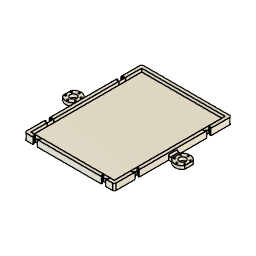
ElevatorAssembly (Autodesk Fusion 360 archive; units mm, degrees)
design "lift_platform"
part number: 2025-09-29-11-11-04-604
Autodesk Fusion 360 part; units mm, degrees
(part 1 of 2)
sketch "Sketch8" plane through (0, 0, 0) normal (0, 0, 1) x (1, 0, 0)
  line L0 (0, 0) -> (256, 0)
  line L1 (256, 0) -> (256, 340)
  line L2 (256, 340) -> (0, 340)
  line L3 (0, 340) -> (0, 0)
  line L4 (0, 340) -> (256, 340)
  line L5 (256, 340) -> (256, 350)
  line L6 (256, 350) -> (0, 350)
  line L7 (0, 350) -> (0, 340)
  line L8 (0, 350) -> (-10, 350)
  line L9 (-10, 350) -> (-10, 0)
  line L10 (-10, 0) -> (0, 0)
  line L11 (0, 0) -> (0, 350)
  line L12 (-10, 0) -> (256, 0)
  line L13 (256, 0) -> (256, -10)
  line L14 (256, -10) -> (-10, -10)
  line L15 (-10, -10) -> (-10, 0)
  line L16 (256, 350) -> (266, 350)
  line L17 (266, 350) -> (266, -10)
  line L18 (266, -10) -> (256, -10)
  line L19 (256, -10) -> (256, 350)
  line L20 (0, 170) -> (256, 170)
  line L21 (256, 170) -> (276, 170)
  line L22 (276, 170) -> (276, 156.885)
  line L23 (276, 156.885) -> (256, 156.885)
  line L24 (256, 156.885) -> (256, 170)
  line L25 (256, 170) -> (276, 170)
  line L26 (276, 170) -> (276, 183.115)
  line L27 (276, 183.115) -> (256, 183.115)
  line L28 (256, 183.115) -> (256, 170)
  line L29 (128, 340) -> (128, 0)
  line L30 (-20, 170) -> (-20, 156.885)
  line L31 (0, 170) -> (-20, 170)
  line L32 (-20, 156.885) -> (0, 156.885)
  line L33 (0, 183.115) -> (0, 170)
  line L34 (-20, 170) -> (-20, 183.115)
  line L35 (0, 170) -> (-20, 170)
  line L36 (0, 156.885) -> (0, 170)
  line L37 (-20, 183.115) -> (0, 183.115)
  dimension "d58" = 340
  dimension "d59" = 256
  dimension "d60" = 10
  dimension "d61" = 10
  dimension "d62" = 10
  dimension "d63" = 10
  dimension "d64" = 20
  dimension "d65" = 13.115
  dimension "d66" = 13.115
  constraint horizontal L0
  constraint vertical L1
  constraint horizontal L2
  constraint vertical L3
  constraint coincident L0.start L3.end
  constraint horizontal L4
  constraint vertical L5
  constraint horizontal L6
  constraint vertical L7
  constraint horizontal L8
  constraint vertical L9
  constraint horizontal L10
  constraint vertical L11
  constraint horizontal L12
  constraint vertical L13
  constraint horizontal L14
  constraint vertical L15
  constraint horizontal L16
  constraint vertical L17
  constraint horizontal L18
  constraint vertical L19
  constraint midpoint L3 L20.start
  constraint midpoint L19 L20.end
  constraint perpendicular L19 L20
  constraint horizontal L21
  constraint vertical L22
  constraint horizontal L23
  constraint vertical L24
  constraint horizontal L25
  constraint vertical L26
  constraint horizontal L27
  constraint vertical L28
  constraint midpoint L2 L29.start
  constraint midpoint L0 L29.end
  constraint symmetric L20.end L29 L20.start
  constraint symmetric L21.end L29 L30.start
  constraint symmetric L22.end L29 L30.end
  constraint symmetric L23.end L29 L32.end
  constraint symmetric L26.end L29 L34.end
  constraint symmetric L27.end L29 L33.start
  measures "d58" distance of L0.start L2.end
  measures "d59" distance of L0.start L0.end
  measures "d60" distance of L2.end L6.end
  measures "d61" distance of L6.end L8.end
  measures "d62" distance of L9.end L14.end
  measures "d63" distance of L5.end L16.end
  measures "d64" distance of L20.end L21.end
  measures "d65" distance of L20.end L23.end
  measures "d66" distance of L20.end L27.end
extrude "Extrude10" add sketch "Sketch8" along normal blind 15 makes body 1
sketch "Sketch9" plane through (0, 0, 15) normal (0, 0, 1) x (-1, 0, 0)
  line L0 (20, -183.115) -> (20, -156.885)
  line L1 (20, -156.885) -> (10, -156.885)
  line L2 (10, -156.885) -> (10, 10)
  line L3 (10, 10) -> (-266, 10)
  line L4 (-266, 10) -> (-266, -156.885)
  line L5 (-266, -156.885) -> (-276, -156.885)
  line L6 (-276, -156.885) -> (-276, -183.115)
  line L7 (-276, -183.115) -> (-266, -183.115)
  line L8 (-266, -183.115) -> (-266, -350)
  line L9 (-266, -350) -> (10, -350)
  line L10 (10, -350) -> (10, -183.115)
  line L11 (10, -183.115) -> (20, -183.115)
  line L12 (-256, -156.885) -> (-256, -170)
  line L13 (-128, 0) -> (-128, -340)
  line L14 (-256, 10) -> (-256, 0)
  line L15 (-266, -340) -> (-256, -340)
  line L16 (0, -340) -> (0, 0)
  line L17 (-256, -340) -> (0, -340)
  line L18 (0, 0) -> (-256, 0)
  line L19 (-266, -340) -> (0, -340)
  line L20 (0, -350) -> (-266, -350)
  line L21 (-256, 0) -> (-256, -340)
  line L22 (-266, -350) -> (-266, -340)
  line L23 (0, -350) -> (0, 10)
  line L24 (-256, -170) -> (-276, -170)
  line L25 (-256, -183.115) -> (-256, -170)
  line L26 (10, 10) -> (10, -350)
  line L27 (-276, -170) -> (-276, -183.115)
  line L28 (-276, -183.115) -> (-256, -183.115)
  line L29 (0, -156.885) -> (0, -170)
  line L30 (10, -350) -> (0, -350)
  line L31 (0, 10) -> (10, 10)
  line L32 (20, -183.115) -> (0, -183.115)
  line L33 (-256, -340) -> (-256, 10)
  line L34 (-276, -156.885) -> (-256, -156.885)
  line L35 (-276, -170) -> (-276, -156.885)
  line L36 (0, 0) -> (0, 10)
  line L37 (0, -183.115) -> (0, -170)
  line L38 (20, -170) -> (20, -156.885)
  line L39 (-266, 10) -> (-266, -340)
  line L40 (-256, 10) -> (-266, 10)
  line L41 (0, -340) -> (0, -350)
  line L42 (0, -170) -> (20, -170)
  line L43 (20, -156.885) -> (0, -156.885)
  line L44 (20, -170) -> (20, -183.115)
  line L45 (-256, -170) -> (-276, -170)
  line L46 (0, -170) -> (20, -170)
  line L47 (-256, -170) -> (0, -170)
  line L48 (-256, 0) -> (0, 0)
  line L49 (0, 10) -> (-256, 10)
  point P0 (-256, -340)
  dimension "d69" = 340
  dimension "d70" = 256
  dimension "d71" = 10
  dimension "d72" = 10
  dimension "d73" = 10
  dimension "d74" = 10
  dimension "d75" = 20
  dimension "d76" = 13.115
  dimension "d77" = 13.115
  constraint horizontal L17
  constraint vertical L16
  constraint horizontal L18
  constraint vertical L21
  constraint coincident P0 L15.end
  constraint horizontal L48
  constraint vertical L36
  constraint horizontal L49
  constraint vertical L14
  constraint horizontal L40
  constraint vertical L39
  constraint horizontal L15
  constraint vertical L33
  constraint horizontal L19
  constraint vertical L41
  constraint horizontal L20
  constraint vertical L22
  constraint horizontal L31
  constraint vertical L26
  constraint horizontal L30
  constraint vertical L23
  constraint midpoint L12.end L21
  constraint midpoint L29.end L23
  constraint perpendicular L23 L47
  constraint horizontal L46
  constraint vertical L44
  constraint horizontal L32
  constraint vertical L37
  constraint horizontal L42
  constraint vertical L38
  constraint horizontal L43
  constraint vertical L29
  constraint midpoint L13.start L18
  constraint midpoint L13.end L17
  constraint symmetric L12.end L29.end L13
  constraint symmetric L24.end L38.start L13
  constraint symmetric L0.start L6.end L13
  constraint symmetric L32.end L25.start L13
  constraint symmetric L38.start L24.end L13
  constraint symmetric L5.end L0.end L13
  constraint symmetric L12.start L29.start L13
  measures "d69" distance of P0 L14.end
  measures "d70" distance of L16.start P0
  measures "d71" distance of L14.end L14.start
  measures "d72" distance of L3.end L14.start
  measures "d73" distance of L15.start L8.end
  measures "d74" distance of L2.end L23.end
  measures "d75" distance of L38.start L29.end
  measures "d76" distance of L32.end L29.end
  measures "d77" distance of L29.start L29.end
extrude "Extrude11" add sketch "Sketch9" along normal blind 10 contours L16 L23 L26 L32 L37 L42 L46 | L9 L10 L16 L23 L26 L30 L32 L41 | L16 L23 L26 L29 L42 L43 L46 | L2 L3 L16 L23 L26 L31 L36 L43 | L8 L9 L15 L17 L19 L20 L22 L23 L41 | L3 L14 L18 L23 L33 L36 L48 L49 | L12 L21 L24 L33 L34 L39 L45 | L21 L24 L25 L28 L33 L39 L45 | L8 L15 L19 L21 L28 L33 L39 | L3 L4 L14 L21 L33 L34 L39 L40 bodies 1
sketch "Sketch10" plane through (0, 0, 15) normal (0, 0, 1) x (-1, 0, 0)
  line L0 (0, -340) -> (0, 0)
  line L1 (0, 0) -> (-256, 0)
  line L2 (-256, 0) -> (-256, -340)
  line L3 (-256, -340) -> (0, -340)
  arc A0 (109.5, -146.8851) -> (70.5, -146.8851) centre (90, -160) ccw
  circle A1 centre (105.1554, -168.75) radius 2.5
  line L4 (109.5, -173.1149) -> (109.5, -146.8851)
  circle A2 centre (90, -160) radius 10
  line L5 (90, -136.5) -> (90, -183.5)
  line L6 (70.5, -146.8851) -> (70.5, -173.1149)
  line L7 (109.5, -173.1149) -> (109.5, -146.8851)
  line L8 (70.5, -146.8851) -> (70.5, -172.6262)
  circle A3 centre (90, -142.5) radius 2.5
  circle A4 centre (74.8446, -151.25) radius 2.5
  circle A5 centre (74.8446, -168.75) radius 2.5
  arc A6 (70.5, -173.1149) -> (109.5, -173.1149) centre (90, -160) ccw
  circle A7 centre (90, -160) radius 11
  circle A8 centre (105.1554, -151.25) radius 2.5
  circle A9 centre (90, -177.5) radius 2.5
  point P0 (90, -160)
  constraint coincident L4.start L7.start
  constraint coincident A0.start L4.end
  constraint coincident A0.end L6.start
  constraint coincident L8.end L6
  constraint midpoint L5.start A0
  constraint midpoint L5.end A6
  constraint concentric A2 A6
extrude "Extrude12" add sketch "Sketch10" along normal blind 15 separate body contours A0 L4 L5 L7 A3 A6 A7 A9 | A0 L5 L6 L8 A3 A6 A7 A9 | A2 L5 A7 | A2 L5 A7 makes body 2
extrude "Extrude13" cut 3 faces at (85.3333, 226.6667, 15) (-13.3333, 165.6283, 15) (269.3333, 174.3717, 15) along direction (0, 0, -1) blind 5 on bodies 1 bodies 1
extrude "Extrude14" cut 1 faces at (262.6667, 226.6667, 25) along direction (0, 0, -1) blind 5 on bodies 1 bodies 1
extrude "Extrude15" cut 1 faces at (-80.6272, 175.6522, 30) along direction (0, 0, -1) blind 5 on bodies 2 bodies 2
copy_body "CopyPasteBodies2" bodies 2 makes body 3
move_body "Move2" bodies 3 to x (1, 0, 0) y (0, 1, 0) z (0, 0, 1) at (440, 0, 0)
move_body "Align1" bodies 2 to x (1, 0, 0) y (0, 1, 0) z (0, 0, 1) at (50.5, 10, -15)
move_body "Align2" bodies 3 to x (1, 0, 0) y (0, 1, 0) z (0, 0, 1) at (-54.5, 10, -15)
fillet "Fillet4" radius 5 4 edges at (-10, -10, 10) (266, -10, 10) (266, 350, 10) (-10, 350, 10) on bodies 1
fillet "Fillet5" radius 5 2 edges at (266, 170, 10) (-10, 170, 10) on bodies 1
sketch "Sketch11" plane through (0, 0, 20) normal (0, 0, 1) x (-1, 0, 0)
  line L0 (0, -340) -> (-256, -340)
  line L1 (-256, -340) -> (-256, 0)
  line L2 (-256, 0) -> (0, 0)
  line L3 (0, 0) -> (0, -340)
  arc A0 (5, -350) -> (10, -345) centre (5, -345) ccw
  line L4 (10, -345) -> (10, 5)
  arc A1 (10, 5) -> (5, 10) centre (5, 5) ccw
  line L5 (5, 10) -> (-261, 10)
  arc A2 (-261, 10) -> (-266, 5) centre (-261, 5) ccw
  line L6 (-266, 5) -> (-266, -345)
  arc A3 (-266, -345) -> (-261, -350) centre (-261, -345) ccw
  line L7 (-261, -350) -> (5, -350)
  line L8 (-128, 10) -> (-128, -350)
  line L9 (-324.6319, -170) -> (70, -170)
  line L10 (-13, 0.0014) -> (-33, 0.0014)
  line L11 (-33, 0.0014) -> (-33, 7)
  line L12 (-33, 0.0014) -> (-33, 7)
  line L13 (-13, 7) -> (-13, 0.0014)
  line L14 (-13, 0.0014) -> (-33, 0.0014)
  line L15 (-13, 7) -> (-13, 0.0014)
  line L16 (-33, 7) -> (-13, 7)
  line L17 (-33, 7) -> (-13, 7)
  line L18 (7, -49.9986) -> (7, -69.9986)
  line L19 (7, -69.9986) -> (0.0014, -69.9986)
  line L20 (7, -69.9986) -> (0.0014, -69.9986)
  line L21 (0.0014, -49.9986) -> (7, -49.9986)
  line L22 (7, -49.9986) -> (7, -69.9986)
  line L23 (0.0014, -49.9986) -> (7, -49.9986)
  line L24 (0.0014, -69.9986) -> (0.0014, -49.9986)
  line L25 (0.0014, -69.9986) -> (0.0014, -49.9986)
  line L26 (-33, 7) -> (-13, 7)
  line L27 (-13, 7) -> (-13, 10)
  line L28 (-13, 10) -> (-33, 10)
  line L29 (-33, 10) -> (-33, 7)
  line L30 (7, -49.9986) -> (10, -49.9986)
  line L31 (10, -49.9986) -> (10, -69.9986)
  line L32 (10, -69.9986) -> (7, -69.9986)
  line L33 (7, -69.9986) -> (7, -49.9986)
  line L34 (-33, 10) -> (-29, 10)
  line L35 (-29, 10) -> (-29, 7)
  line L36 (-29, 7) -> (-33, 7)
  line L37 (-33, 7) -> (-33, 10)
  line L38 (-13, 10) -> (-17, 10)
  line L39 (-17, 10) -> (-17, 7)
  line L40 (-17, 7) -> (-13, 7)
  line L41 (-13, 7) -> (-13, 10)
  line L42 (10, -49.9986) -> (7, -49.9986)
  line L43 (7, -49.9986) -> (7, -53.9986)
  line L44 (7, -53.9986) -> (10, -53.9986)
  line L45 (10, -53.9986) -> (10, -49.9986)
  line L46 (7, -69.9986) -> (10, -69.9986)
  line L47 (10, -69.9986) -> (10, -65.9986)
  line L48 (10, -65.9986) -> (7, -65.9986)
  line L49 (7, -65.9986) -> (7, -69.9986)
  line L50 (-263, -69.9986) -> (-256.0014, -69.9986)
  line L51 (-263, -69.9986) -> (-256.0014, -69.9986)
  line L52 (-256.0014, -49.9986) -> (-263, -49.9986)
  line L53 (-263, -49.9986) -> (-263, -69.9986)
  line L54 (-256.0014, -49.9986) -> (-263, -49.9986)
  line L55 (-256.0014, -69.9986) -> (-256.0014, -49.9986)
  line L56 (-256.0014, -69.9986) -> (-256.0014, -49.9986)
  line L57 (-263, -65.9986) -> (-263, -69.9986)
  line L58 (-263, -49.9986) -> (-263, -69.9986)
  line L59 (-266, -69.9986) -> (-266, -65.9986)
  line L60 (-263, -49.9986) -> (-263, -53.9986)
  line L61 (-266, -69.9986) -> (-263, -69.9986)
  line L62 (-263, -53.9986) -> (-266, -53.9986)
  line L63 (-266, -53.9986) -> (-266, -49.9986)
  line L64 (-266, -65.9986) -> (-263, -65.9986)
  line L65 (-263, -69.9986) -> (-266, -69.9986)
  line L66 (-266, -49.9986) -> (-266, -69.9986)
  line L67 (-266, -49.9986) -> (-263, -49.9986)
  line L68 (-263, -69.9986) -> (-263, -49.9986)
  line L69 (-263, -49.9986) -> (-266, -49.9986)
  line L70 (-223, 10) -> (-227, 10)
  line L71 (-227, 10) -> (-227, 7)
  line L72 (-239, 10) -> (-239, 7)
  line L73 (-239, 7) -> (-243, 7)
  line L74 (-243, 10) -> (-223, 10)
  line L75 (-223, 7) -> (-243, 7)
  line L76 (-243, 10) -> (-239, 10)
  line L77 (-227, 7) -> (-223, 7)
  line L78 (-243, 7) -> (-243, 0.0014)
  line L79 (-243, 7) -> (-243, 0.0014)
  line L80 (-223, 7) -> (-243, 7)
  line L81 (-243, 7) -> (-243, 10)
  line L82 (-223, 10) -> (-223, 7)
  line L83 (-243, 0.0014) -> (-223, 0.0014)
  line L84 (-223, 0.0014) -> (-223, 7)
  line L85 (-243, 7) -> (-243, 10)
  line L86 (-223, 7) -> (-223, 10)
  line L87 (-243, 0.0014) -> (-223, 0.0014)
  line L88 (-223, 0.0014) -> (-223, 7)
  line L89 (-223, 7) -> (-243, 7)
  line L90 (-243, -347) -> (-243, -340.0014)
  line L91 (-263, -270.0014) -> (-266, -270.0014)
  line L92 (-263, -290.0014) -> (-266, -290.0014)
  line L93 (-17, -347) -> (-13, -347)
  line L94 (-256.0014, -270.0014) -> (-256.0014, -290.0014)
  line L95 (-263, -290.0014) -> (-263, -286.0014)
  line L96 (-266, -286.0014) -> (-266, -290.0014)
  line L97 (-227, -347) -> (-223, -347)
  line L98 (-243, -347) -> (-243, -340.0014)
  line L99 (-223, -347) -> (-243, -347)
  line L100 (10, -290.0014) -> (7, -290.0014)
  line L101 (-13, -350) -> (-17, -350)
  line L102 (-243, -350) -> (-239, -350)
  line L103 (-263, -290.0014) -> (-263, -270.0014)
  line L104 (-263, -286.0014) -> (-266, -286.0014)
  line L105 (-243, -347) -> (-243, -350)
  line L106 (-33, -347) -> (-13, -347)
  line L107 (-239, -350) -> (-239, -347)
  line L108 (-239, -347) -> (-243, -347)
  line L109 (-13, -340.0014) -> (-33, -340.0014)
  line L110 (-13, -347) -> (-13, -340.0014)
  line L111 (7, -290.0014) -> (7, -270.0014)
  arc A4 (5, -350) -> (10, -345) centre (5, -345) ccw
  line L112 (7, -290.0014) -> (10, -290.0014)
  line L113 (-223, -340.0014) -> (-223, -347)
  line L114 (-223, -350) -> (-227, -350)
  line L115 (10, -270.0014) -> (10, -274.0014)
  line L116 (-13, -347) -> (-13, -350)
  line L117 (-33, -340.0014) -> (-33, -347)
  line L118 (7, -270.0014) -> (10, -270.0014)
  line L119 (-13, -347) -> (-13, -350)
  line L120 (7, -286.0014) -> (10, -286.0014)
  line L121 (-29, -350) -> (-29, -347)
  line L122 (-266, -270.0014) -> (-266, -274.0014)
  arc A5 (-266, -345) -> (-261, -350) centre (-261, -345) ccw
  line L123 (10, -290.0014) -> (10, -270.0014)
  line L124 (7, -270.0014) -> (7, -290.0014)
  line L125 (-13, -350) -> (-33, -350)
  line L126 (-243, -350) -> (-223, -350)
  line L127 (-256.0014, -270.0014) -> (-256.0014, -290.0014)
  line L128 (-266, -290.0014) -> (-263, -290.0014)
  line L129 (-33, -350) -> (-29, -350)
  line L130 (-13, -347) -> (-13, -340.0014)
  line L131 (7, -290.0014) -> (7, -286.0014)
  line L132 (-223, -347) -> (-243, -347)
  line L133 (-263, -274.0014) -> (-263, -270.0014)
  line L134 (-263, -290.0014) -> (-263, -270.0014)
  line L135 (-223, -347) -> (-243, -347)
  line L136 (-227, -350) -> (-227, -347)
  line L137 (-243, -340.0014) -> (-223, -340.0014)
  line L138 (-33, -347) -> (-13, -347)
  line L139 (10, -270.0014) -> (7, -270.0014)
  line L140 (-33, -340.0014) -> (-33, -347)
  line L141 (-29, -347) -> (-33, -347)
  line L142 (-33, -350) -> (-33, -347)
  line L143 (-263, -270.0014) -> (-263, -290.0014)
  line L144 (-243, -340.0014) -> (-223, -340.0014)
  line L145 (-266, -290.0014) -> (-266, -270.0014)
  line L146 (10, -274.0014) -> (7, -274.0014)
  line L147 (10, -286.0014) -> (10, -290.0014)
  line L148 (-33, -347) -> (-33, -350)
  line L149 (-243, -347) -> (-243, -350)
  line L150 (-266, -274.0014) -> (-263, -274.0014)
  line L151 (-266, -270.0014) -> (-263, -270.0014)
  line L152 (0.0014, -270.0014) -> (0.0014, -290.0014)
  line L153 (-223, -340.0014) -> (-223, -347)
  line L154 (-33, -347) -> (-13, -347)
  line L155 (-223, -347) -> (-223, -350)
  line L156 (0.0014, -270.0014) -> (0.0014, -290.0014)
  line L157 (-256.0014, -290.0014) -> (-263, -290.0014)
  line L158 (-223, -350) -> (-223, -347)
  line L159 (7, -274.0014) -> (7, -270.0014)
  line L160 (-13, -340.0014) -> (-33, -340.0014)
  line L161 (7, -290.0014) -> (7, -270.0014)
  line L162 (-17, -350) -> (-17, -347)
  line L163 (-263, -270.0014) -> (-256.0014, -270.0014)
  line L164 (-256, -340) -> (0, -340)
  line L165 (0.0014, -290.0014) -> (7, -290.0014)
  line L166 (0.0014, -290.0014) -> (7, -290.0014)
  line L167 (5, -350) -> (-261, -350)
  line L168 (7, -270.0014) -> (0.0014, -270.0014)
  line L169 (-263, -270.0014) -> (-256.0014, -270.0014)
  line L170 (7, -270.0014) -> (0.0014, -270.0014)
  line L171 (-256.0014, -290.0014) -> (-263, -290.0014)
  point P0 (-128, -350)
  point P1 (0, -340)
  dimension "d92" = 4
  dimension "d93" = 4
  constraint midpoint L5 L8.start
  constraint midpoint L7 P0
  constraint perpendicular L4 L9
  constraint horizontal L10
  constraint vertical L12
  constraint horizontal L16
  constraint vertical L13
  constraint horizontal L14
  constraint vertical L11
  constraint horizontal L17
  constraint vertical L15
  constraint horizontal L26
  constraint vertical L27
  constraint horizontal L28
  constraint vertical L29
  constraint coincident L5 L27.end
  constraint horizontal L30
  constraint vertical L31
  constraint horizontal L32
  constraint vertical L33
  constraint coincident L4 L31.end
  constraint horizontal L34
  constraint vertical L35
  constraint horizontal L36
  constraint vertical L37
  constraint coincident L16 L35.end
  constraint horizontal L38
  constraint vertical L39
  constraint horizontal L40
  constraint vertical L41
  constraint coincident L26 L39.end
  constraint horizontal L42
  constraint vertical L43
  constraint horizontal L44
  constraint vertical L45
  constraint horizontal L46
  constraint vertical L47
  constraint horizontal L48
  constraint vertical L49
  constraint symmetric L8 L10.start L78.end
  constraint symmetric L8 L13.start L73.end
  constraint symmetric L8 L11.end L75.start
  constraint symmetric L8 L10.end L83.end
  constraint symmetric L8 L18.start L52.end
  constraint symmetric L8 L21.start L52.start
  constraint symmetric L8 L19.end L50.end
  constraint symmetric L8 L18.end L50.start
  constraint symmetric L8 L27.end L74.start
  constraint symmetric L8 L28.end L70.start
  constraint symmetric L8 L30.end L63.end
  constraint symmetric L8 L31.end L59.start
  constraint symmetric L8 L34.end L70.end
  constraint symmetric L8 L35.end L71.end
  constraint symmetric L8 L38.end L72.start
  constraint symmetric L8 L39.end L72.end
  constraint symmetric L8 L43.end L60.end
  constraint symmetric L8 L44.end L62.end
  constraint symmetric L8 L47.end L59.end
  constraint symmetric L8 L48.end L57.start
  constraint symmetric L2.end L9 P1
  constraint symmetric L1.end L9 L0.end
  constraint symmetric L4.end L9 A0.end
  constraint symmetric A1.end L9 A0.start
  constraint symmetric A1 L9 A4
  constraint symmetric L5.end L9 A3.end
  constraint symmetric A2.end L9 L6.end
  constraint symmetric A2 L9 A5
  constraint symmetric L8.start L9 P0
  constraint symmetric L9 L10.start L109.start
  constraint symmetric L9 L13.start L93.end
  constraint symmetric L9 L11.end L106.start
  constraint symmetric L9 L10.end L109.end
  constraint symmetric L9 L18.start L100.end
  constraint symmetric L9 L21.start L152.end
  constraint symmetric L9 L19.end L152.start
  constraint symmetric L9 L18.end L111.end
  constraint symmetric L9 L27.end L101.start
  constraint symmetric L9 L28.end L125.end
  constraint symmetric L9 L30.end L100.start
  constraint symmetric L9 L31.end L115.start
  constraint symmetric L9 L34.end L121.start
  constraint symmetric L9 L35.end L121.end
  constraint symmetric L9 L38.end L101.end
  constraint symmetric L9 L39.end L93.start
  constraint symmetric L9 L43.end L120.start
  constraint symmetric L9 L44.end L120.end
  constraint symmetric L9 L47.end L115.end
  constraint symmetric L9 L48.end L146.end
  constraint symmetric L9 L50.end L94.start
  constraint symmetric L9 L52.end L92.start
  constraint symmetric L9 L59.start L91.end
  constraint symmetric L9 L52.start L94.end
  constraint symmetric L9 L50.start L91.start
  constraint symmetric L9 L63.end L92.end
  constraint symmetric L9 L60.end L95.end
  constraint symmetric L9 L59.end L122.end
  constraint symmetric L9 L57.start L133.start
  constraint symmetric L9 L62.end L96.start
  constraint symmetric L9 L73.end L90.start
  constraint symmetric L9 L78.end L90.end
  constraint symmetric L9 L74.start L102.start
  constraint symmetric L9 L83.end L113.start
  constraint symmetric L9 L70.start L114.start
  constraint symmetric L9 L71.end L97.start
  constraint symmetric L9 L75.start L97.end
  constraint symmetric L9 L72.end L107.end
  constraint symmetric L9 L72.start L102.end
  constraint symmetric L9 L70.end L114.end
  measures "d92" distance of L30.end L44.end
  measures "d93" distance of L18.end L48.end
extrude "Extrude16" cut sketch "Sketch11" against normal blind 20 contours L4 L111 L120 L123 L124 L146 L161 | L111 L124 L131 L152 L156 L159 L161 L165 L166 L168 L170 | L4 L18 L22 L31 L33 L44 L48 | L18 L19 L20 L21 L22 L23 L24 L25 L33 L43 L49 | L6 L53 L58 L62 L64 L66 L68 | L50 L51 L52 L53 L54 L55 L56 L57 L58 L60 L68 | L6 L103 L104 L134 L143 L145 L150 | L94 L95 L103 L127 L133 L134 L143 L157 L163 L169 L171 | L5 L16 L17 L26 L28 L35 L39 | L10 L11 L12 L13 L14 L15 L16 L17 L26 L36 L40 | L5 L71 L72 L74 L75 L80 L89 | L73 L75 L77 L78 L79 L80 L83 L84 L87 L88 L89 bodies 1

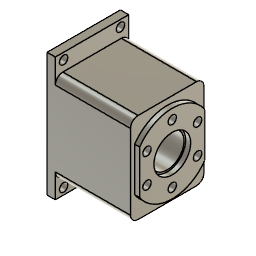
design "MotorCasing"
part number: 2025-09-29-15-38-35-951
Autodesk Fusion 360 part; units mm, degrees
sketch "Sketch1" plane through (0, 0, 0) normal (1, 0, 0) x (0, 1, 0)
  circle A0 centre (0, 32.5) radius 2.5
  arc A1 (-19.5, 36.8851) -> (19.5, 36.8851) centre (0, 50) ccw
  circle A2 centre (15.1554, 58.75) radius 2.5
  circle A3 centre (0, 67.5) radius 2.5
  circle A4 centre (0, 50) radius 10
  line L0 (19.5, 36.8851) -> (19.5, 63.1149)
  circle A5 centre (15.1554, 41.25) radius 2.5
  line L1 (-19.5, 63.1149) -> (-19.5, 36.8851)
  arc A6 (19.5, 63.1149) -> (-19.5, 63.1149) centre (0, 50) ccw
  line L2 (19.5, 36.8851) -> (19.5, 63.1149)
  circle A7 centre (-15.1554, 58.75) radius 2.5
  circle A8 centre (0, 50) radius 11
  line L3 (0, 73.5) -> (0, 26.5)
  line L4 (-19.5, 63.1149) -> (-19.5, 37.3738)
  circle A9 centre (-15.1554, 41.25) radius 2.5
  line L5 (0, 50) -> (-22, 50)
  line L6 (-22, 50) -> (-22, 23)
  line L7 (-22, 23) -> (0, 23)
  line L8 (0, 23) -> (0, 50)
  circle A10 centre (15.1554, 41.25) radius 2.5
  circle A11 centre (0, 32.5) radius 2.5
  line L9 (0, 23) -> (0, 50)
  line L10 (22, 23) -> (0, 23)
  line L11 (0, 50) -> (22, 50)
  line L12 (22, 50) -> (22, 23)
  line L13 (-22, 50) -> (-22, 77)
  line L14 (0, 50) -> (-22, 50)
  line L15 (-22, 77) -> (0, 77)
  line L16 (0, 77) -> (0, 50)
  line L17 (22, 77) -> (0, 77)
  circle A12 centre (0, 67.5) radius 2.5
  line L18 (22, 50) -> (22, 77)
  line L19 (0, 77) -> (0, 50)
  line L20 (0, 50) -> (22, 50)
  arc A13 (19.5, 63.1149) -> (-19.5, 63.1149) centre (0, 50) ccw
  circle A14 centre (0, 67.5) radius 2.5
  circle A15 centre (15.1554, 58.75) radius 2.5
  circle A16 centre (15.1554, 58.75) radius 2.5
  circle A17 centre (-15.1554, 58.75) radius 2.5
  point P0 (0, 50)
  point P1 (0, 50)
  point P2 (0, 26.5)
  point P3 (19.5, 37.3738)
  point P4 (0, 50)
  point P5 (19.5, 36.8851)
  point P6 (0, 50)
  point P7 (0, 73.5)
  point P8 (0, 50)
  point P9 (0, 50)
  point P10 (0, 73.5)
  point P11 (19.5, 63.1149)
  point P12 (-19.5, 62.6262)
  point P13 (0, 50)
  point P14 (19.5, 62.6262)
  point P15 (19.5, 63.1149)
  point P16 (0, 50)
  point P17 (0, 50)
  constraint coincident P5 A1.end
  constraint coincident P15 P11
  constraint coincident L1.start A6.end
  constraint coincident L4.end L1
  constraint midpoint P10 A6
  constraint midpoint P2 A1
  constraint concentric A1 A4
  constraint horizontal L5
  constraint vertical L6
  constraint horizontal L7
  constraint vertical L8
  constraint coincident P17 P16
  constraint symmetric P17 L3 P16
  constraint symmetric A1.start L3 P5
  constraint symmetric P2 L3 L3.end
  constraint symmetric L4.end L3 P3
  constraint symmetric A0 L3 A11
  constraint symmetric L3 A9 A10
  constraint symmetric L3 P17 P16
  constraint symmetric L3 L5.end L11.end
  constraint symmetric L3 L6.end L10.start
  constraint symmetric L3 L7.end L8.start
  constraint symmetric P17 L11 P16
  constraint symmetric A1.start L11 L1.start
  constraint symmetric P5 L11 P15
  constraint symmetric P2 L11 P10
  constraint symmetric L4.end L11 P12
  constraint symmetric A0 L11 A14
  constraint symmetric A1 L11 A13
  constraint symmetric A5 L11 A16
  constraint symmetric A9 L11 A17
  constraint symmetric L5.end L11 L6.start
  constraint symmetric L6.end L11 L13.end
  constraint symmetric L7.end L11 L15.end
  constraint symmetric L12.start L11 L18.start
  constraint symmetric P3 L11 P14
  constraint symmetric L10.start L11 L17.start
  constraint symmetric A10 L11 A15
  constraint symmetric A11 L11 A12
extrude "Extrude1" add sketch "Sketch1" along normal blind 50 contours A0 A1 L0 L2 A8 L3 L8 A11 L9 L11 L20 | A0 A1 L1 A8 L3 L4 L5 L8 A11 L9 L14 | A4 A8 L3 L8 L9 L11 L20 | A4 A8 L3 L5 L8 L9 L14 | A1 L1 L4 L5 L6 L7 L8 L9 L14 | A1 L0 L2 L8 L9 L10 L11 L12 L20 | A3 L1 A6 A8 L3 L4 L5 L14 L16 A12 L19 A13 A14 | A4 A8 L3 L5 L14 L16 L19 | A4 A8 L3 L11 L16 L19 L20 | A3 L0 A6 L2 A8 L3 L11 L16 A12 L19 L20 A13 A14 | L1 A6 L4 L5 L13 L14 L15 L16 L19 A13 | L0 A6 L2 L11 L16 L17 L18 L19 L20 A13
sketch "Sketch2" plane through (50, 0, 0) normal (1, 0, 0) x (0, 1, 0)
  circle A0 centre (0, 32.5) radius 2.5
  circle A1 centre (-15.1554, 58.75) radius 2.5
  circle A2 centre (-15.1554, 41.25) radius 2.5
  circle A3 centre (0, 50) radius 10
  circle A4 centre (15.1554, 58.75) radius 2.5
  circle A5 centre (15.1554, 41.25) radius 2.5
  circle A6 centre (0, 67.5) radius 2.5
  line L0 (22, 23) -> (22, 77)
  line L1 (22, 77) -> (-22, 77)
  line L2 (-22, 77) -> (-22, 23)
  line L3 (-22, 23) -> (22, 23)
  circle A7 centre (0, 32.5) radius 2.5
  arc A8 (-19.5, 36.8851) -> (19.5, 36.8851) centre (0, 50) ccw
  circle A9 centre (15.1554, 58.75) radius 2.5
  circle A10 centre (0, 67.5) radius 2.5
  circle A11 centre (0, 50) radius 10
  line L4 (19.5, 36.8851) -> (19.5, 63.1149)
  circle A12 centre (15.1554, 41.25) radius 2.5
  line L5 (-19.5, 63.1149) -> (-19.5, 36.8851)
  arc A13 (19.5, 63.1149) -> (-19.5, 63.1149) centre (0, 50) ccw
  line L6 (19.5, 36.8851) -> (19.5, 63.1149)
  circle A14 centre (-15.1554, 58.75) radius 2.5
  circle A15 centre (0, 50) radius 11
  line L7 (0, 73.5) -> (0, 26.5)
  line L8 (-19.5, 63.1149) -> (-19.5, 37.3738)
  circle A16 centre (-15.1554, 41.25) radius 2.5
  point P0 (0, 50)
  constraint coincident A8.end L4.start
  constraint coincident L4.end A13.start
  constraint coincident L5.start A13.end
  constraint coincident L8.end L5
  constraint midpoint L7.start A13
  constraint midpoint L7.end A8
  constraint concentric A8 A11
extrude "Extrude2" add sketch "Sketch2" along normal blind 3 contours A0 A6 A7 A8 A10 L4 A13 L6 A15 L7 | A0 A6 A7 A8 A10 L5 A13 A15 L7 L8
sketch "Sketch3" plane through (0, 0, 77) normal (0, 0, 1) x (-1, 0, 0)
  line L0 (0, -22) -> (0, 22)
  line L1 (0, 22) -> (-50, 22)
  line L2 (-50, 22) -> (-50, -22)
  line L3 (-50, -22) -> (0, -22)
  line L4 (0, -22) -> (-5, -22)
  line L5 (-5, -22) -> (-5, 22)
  line L6 (-5, 22) -> (0, 22)
  line L7 (0, 22) -> (0, -22)
  dimension "d5" = 5
  constraint horizontal L4
  constraint vertical L5
  constraint horizontal L6
  constraint vertical L7
  constraint coincident L0.start L3.end
  measures "d5" distance of L0.start L4.end
extrude "Extrude3" add sketch "Sketch3" along normal blind 10 contours L0 L1 L3 L4 L5 L6 L7
sketch "Sketch4" plane through (0, 0, 23) normal (0, 0, -1) x (1, 0, 0)
  line L0 (0, 22) -> (0, -22)
  line L1 (0, -22) -> (50, -22)
  line L2 (50, -22) -> (50, 22)
  line L3 (50, 22) -> (0, 22)
  line L4 (0, -22) -> (5, -22)
  line L5 (5, -22) -> (5, 22)
  line L6 (5, 22) -> (0, 22)
  line L7 (0, 22) -> (0, -22)
  dimension "d8" = 5
  constraint horizontal L4
  constraint vertical L5
  constraint horizontal L6
  constraint vertical L7
  constraint coincident L0.end L1.start
  measures "d8" distance of L0.end L4.end
extrude "Extrude4" add sketch "Sketch4" along normal blind 10 contours L0 L1 L3 L4 L5 L6 L7
sketch "Sketch5" plane through (5, 0, 0) normal (1, 0, 0) x (0, 1, 0)
  line L0 (-22, 77) -> (22, 77)
  line L1 (22, 77) -> (22, 87)
  line L2 (22, 87) -> (-22, 87)
  line L3 (-22, 87) -> (-22, 77)
  circle A0 centre (-17, 83) radius 2.5
  circle A1 centre (17, 83) radius 2.5
  circle A2 centre (-17, 17) radius 2.5
  circle A3 centre (17, 17) radius 2.5
  line L4 (22, 13) -> (-22, 13)
  line L5 (-22, 23) -> (-22, 13)
  line L6 (22, 23) -> (22, 13)
  dimension "d11" = 5
  dimension "d12" = 5
  dimension "d13" = 5
  dimension "d14" = 5
  dimension "d15" = 4
  dimension "d16" = 4
  dimension "d17" = 5
  dimension "d18" = 5
  dimension "d19" = 5
  dimension "d20" = 5
  dimension "d21" = 4
  dimension "d22" = 4
  measures "d11" diameter of A0
  measures "d12" diameter of A1
  measures "d13" diameter of A2
  measures "d14" diameter of A3
  measures "d15" distance of A2.centre L4
  measures "d16" distance of A3.centre L4
  measures "d17" distance of A2.centre L5
  measures "d18" distance of A3.centre L6
  measures "d19" distance of L1 A1.centre
  measures "d20" distance of L3 A0.centre
  measures "d21" distance of L2 A0.centre
  measures "d22" distance of L2 A1.centre
extrude "Extrude5" cut sketch "Sketch5" against normal blind 10 contours A0 | A1 | A2 | A3
fillet "Fillet1" radius 4.5 4 edges at (27.5, -22, 77) (27.5, 22, 77) (27.5, 22, 23) (27.5, -22, 23)

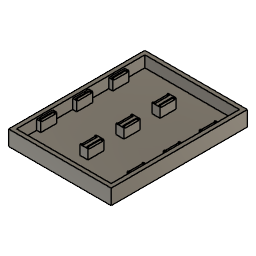
design "Machine1Tray"
part number: 2025-09-29-14-30-21-677
Autodesk Fusion 360 part; units mm, degrees
sketch "Sketch1" plane through (0, 0, 0) normal (0, 0, 1) x (1, 0, 0)
  line L0 (0, 0) -> (236, 0)
  line L1 (236, 0) -> (236, 320)
  line L2 (236, 320) -> (0, 320)
  line L3 (0, 320) -> (0, 0)
  line L4 (0, 0) -> (236, 0)
  line L5 (236, 0) -> (236, -10)
  line L6 (236, -10) -> (0, -10)
  line L7 (0, -10) -> (0, 0)
  line L8 (0, 320) -> (-10, 320)
  line L9 (-10, 320) -> (-10, 0)
  line L10 (-10, 0) -> (0, 0)
  line L11 (0, 0) -> (0, 320)
  line L12 (236, 0) -> (246, 0)
  line L13 (246, 0) -> (246, 320)
  line L14 (246, 320) -> (236, 320)
  line L15 (236, 320) -> (236, 0)
  line L16 (-10, 320) -> (246, 320)
  line L17 (246, 320) -> (246, 330)
  line L18 (246, 330) -> (-10, 330)
  line L19 (-10, 330) -> (-10, 320)
  line L20 (0, 0) -> (-10, 0)
  line L21 (-10, 0) -> (-10, -10)
  line L22 (-10, -10) -> (0, -10)
  line L23 (0, -10) -> (0, 0)
  line L24 (236, 0) -> (246, 0)
  line L25 (246, 0) -> (246, -10)
  line L26 (246, -10) -> (236, -10)
  line L27 (236, -10) -> (236, 0)
  dimension "d1" = 236
  dimension "d2" = 320
  dimension "d3" = 236
  dimension "d4" = 10
  dimension "d5" = 10
  dimension "d6" = 320
  dimension "d7" = 10
  dimension "d8" = 320
  dimension "d9" = 10
  constraint horizontal L0
  constraint vertical L1
  constraint horizontal L2
  constraint vertical L3
  constraint coincident L0.start L3.end
  constraint horizontal L4
  constraint vertical L5
  constraint horizontal L6
  constraint vertical L7
  constraint horizontal L8
  constraint vertical L9
  constraint horizontal L10
  constraint vertical L11
  constraint horizontal L12
  constraint vertical L13
  constraint horizontal L14
  constraint vertical L15
  constraint horizontal L16
  constraint vertical L17
  constraint horizontal L18
  constraint vertical L19
  constraint horizontal L20
  constraint vertical L21
  constraint horizontal L22
  constraint vertical L23
  constraint horizontal L24
  constraint vertical L25
  constraint horizontal L26
  constraint vertical L27
  measures "d1" distance of L0.start L0.end
  measures "d2" distance of L0.start L2.end
  measures "d3" distance of L0.start L0.end
  measures "d4" distance of L0.start L6.end
  measures "d5" distance of L2.end L8.end
  measures "d6" distance of L2.end L0.start
  measures "d7" distance of L0.end L12.end
  measures "d8" distance of L0.end L1.end
  measures "d9" distance of L8.end L18.end
extrude "Extrude1" add sketch "Sketch1" along normal blind 10
sketch "Sketch2" plane through (0, 0, 10) normal (0, 0, 1) x (-1, 0, 0)
  line L0 (-246, 10) -> (-246, -330)
  line L1 (-246, -330) -> (10, -330)
  line L2 (10, -330) -> (10, 10)
  line L3 (10, 10) -> (-246, 10)
  line L4 (10, -330) -> (0, -330)
  line L5 (0, -330) -> (0, 10)
  line L6 (0, 10) -> (10, 10)
  line L7 (10, 10) -> (10, -330)
  line L8 (10, 0) -> (-246, 0)
  line L9 (-246, 0) -> (-246, 10)
  line L10 (-246, 10) -> (10, 10)
  line L11 (10, 10) -> (10, 0)
  line L12 (-246, 10) -> (-236, 10)
  line L13 (-236, 10) -> (-236, -330)
  line L14 (-236, -330) -> (-246, -330)
  line L15 (-246, -330) -> (-246, 10)
  line L16 (10, -330) -> (-246, -330)
  line L17 (-246, -330) -> (-246, -320)
  line L18 (-246, -320) -> (10, -320)
  line L19 (10, -320) -> (10, -330)
  dimension "d12" = 10
  dimension "d13" = 10
  constraint horizontal L4
  constraint vertical L5
  constraint horizontal L6
  constraint vertical L7
  constraint coincident L3 L5.end
  constraint coincident L1.end L2.start
  constraint horizontal L8
  constraint vertical L9
  constraint horizontal L10
  constraint vertical L11
  constraint coincident L0.start L3.end
  constraint coincident L7 L8.start
  constraint horizontal L12
  constraint vertical L13
  constraint horizontal L14
  constraint vertical L15
  constraint horizontal L16
  constraint vertical L17
  constraint horizontal L18
  constraint vertical L19
  measures "d12" distance of L0.start L12.end
  measures "d13" distance of L1.end L18.end
extrude "Extrude2" add sketch "Sketch2" along normal blind 28 contours L0 L3 L8 L9 L10 L12 L13 L15 | L0 L8 L13 L15 L18 | L3 L5 L8 L10 L13 | L0 L1 L13 L14 L15 L16 L17 L18 | L2 L3 L5 L6 L7 L8 L10 L11 | L1 L5 L13 L16 L18 | L2 L5 L7 L8 L18 | L1 L2 L4 L5 L7 L16 L18 L19
sketch "Sketch3" plane through (0, 0, 10) normal (0, 0, 1) x (-1, 0, 0)
  line L0 (-236, -320) -> (0, -320)
  line L1 (0, -320) -> (0, 0)
  line L2 (0, 0) -> (-236, 0)
  line L3 (-236, 0) -> (-236, -320)
  line L4 (0, -50) -> (-118, -50)
  line L5 (-118, -50) -> (-118, -90)
  line L6 (-118, -90) -> (0, -90)
  line L7 (0, -90) -> (0, -50)
  line L8 (-118, -140) -> (-118, -180)
  line L9 (0, -180) -> (0, -140)
  line L10 (0, -140) -> (-118, -140)
  line L11 (-118, -180) -> (0, -180)
  line L12 (-118, -230) -> (-118, -270)
  line L13 (0, -270) -> (0, -230)
  line L14 (0, -230) -> (-118, -230)
  line L15 (-118, -270) -> (0, -270)
  line L16 (-118, -50) -> (-118, -90)
  line L17 (0, -90) -> (0, -50)
  line L18 (0, -50) -> (-118, -50)
  line L19 (-118, -90) -> (0, -90)
  line L20 (-118, -270) -> (-236, -270)
  line L21 (-236, -270) -> (-236, -230)
  line L22 (-236, -230) -> (-118, -230)
  line L23 (-118, -230) -> (-118, -270)
  line L24 (-118, -180) -> (-236, -180)
  line L25 (-236, -180) -> (-236, -140)
  line L26 (-236, -140) -> (-118, -140)
  line L27 (-118, -140) -> (-118, -180)
  line L28 (-118, -90) -> (-236, -90)
  line L29 (-236, -90) -> (-236, -50)
  line L30 (-236, -50) -> (-118, -50)
  line L31 (-118, -50) -> (-118, -90)
  dimension "d16" = 118
  dimension "d17" = 40
  dimension "d18" = 118
  dimension "d19" = 40
  dimension "d20" = 118
  dimension "d21" = 40
  dimension "d22" = 118
  dimension "d23" = 40
  dimension "d24" = 50
  dimension "d25" = 50
  dimension "d26" = 50
  dimension "d27" = 50
  dimension "d28" = 40
  constraint horizontal L4
  constraint vertical L5
  constraint horizontal L6
  constraint vertical L7
  constraint coincident L1 L4.start
  constraint horizontal L10
  constraint vertical L8
  constraint horizontal L11
  constraint vertical L9
  constraint horizontal L14
  constraint vertical L12
  constraint horizontal L15
  constraint vertical L13
  constraint horizontal L18
  constraint vertical L16
  constraint horizontal L19
  constraint vertical L17
  constraint horizontal L20
  constraint vertical L21
  constraint horizontal L22
  constraint vertical L23
  constraint coincident L3 L21.end
  constraint horizontal L24
  constraint vertical L25
  constraint horizontal L26
  constraint vertical L27
  constraint coincident L3 L25.end
  constraint horizontal L28
  constraint vertical L29
  constraint horizontal L30
  constraint vertical L31
  constraint coincident L3 L29.end
  measures "d16" distance of L4.start L4.end
  measures "d17" distance of L4.start L6.end
  measures "d18" distance of L9.end L8.start
  measures "d19" distance of L9.end L9.start
  measures "d20" distance of L13.end L12.start
  measures "d21" distance of L13.end L13.start
  measures "d22" distance of L4.start L4.end
  measures "d23" distance of L4.start L6.end
  measures "d24" distance of L2 L4
  measures "d25" distance of L0 L15
  measures "d26" distance of L11 L14
  measures "d27" distance of L10 L19
  measures "d28" distance of L12.end L12.start
extrude "Extrude3" add sketch "Sketch3" along normal blind 22 contours L3 L12 L20 L21 L22 L23 | L1 L12 L13 L14 L15 L23 | L3 L8 L24 L25 L26 L27 | L1 L8 L9 L10 L11 L27 | L3 L5 L16 L28 L29 L30 L31 | L1 L4 L5 L6 L7 L16 L17 L18 L19 L31
sketch "Sketch4" plane through (0, 0, 32) normal (0, 0, 1) x (-1, 0, 0)
  line L0 (-236, -180) -> (0, -180)
  line L1 (0, -180) -> (0, -140)
  line L2 (0, -140) -> (-236, -140)
  line L3 (-236, -140) -> (-236, -180)
  line L4 (35.6076, 60.8839) -> (35.6076, 66.8839)
  line L5 (35.6076, 66.8839) -> (69.6076, 66.8839)
  line L6 (32.6076, 60.8839) -> (35.6076, 60.8839)
  line L7 (69.6076, 60.8839) -> (35.6076, 60.8839)
  line L8 (32.6076, 60.8839) -> (32.6076, 70.8839)
  line L9 (32.6076, 70.8839) -> (72.6076, 70.8839)
  line L10 (69.6076, 66.8839) -> (69.6076, 60.8839)
  line L11 (35.6076, 66.8839) -> (69.6076, 66.8839)
  line L12 (35.6076, 60.8839) -> (35.6076, 66.8839)
  line L13 (69.6076, 66.8839) -> (69.6076, 60.8839)
  line L14 (72.6076, 60.8839) -> (32.6076, 60.8839)
  line L15 (72.6076, 70.8839) -> (72.6076, 60.8839)
  line L16 (69.6076, 60.8839) -> (72.6076, 60.8839)
  line L17 (72.6076, 60.8839) -> (72.6076, 70.8839)
  line L18 (72.6076, 70.8839) -> (32.6076, 70.8839)
  line L19 (32.6076, 70.8839) -> (32.6076, 60.8839)
  line L20 (0, -90) -> (-10, -90)
  line L21 (-10, -90) -> (-10, -50)
  line L22 (-10, -50) -> (0, -50)
  line L23 (0, -50) -> (0, -90)
  line L24 (-10, -87) -> (-4, -87)
  line L25 (-4, -87) -> (-4, -53)
  line L26 (-4, -53) -> (-10, -53)
  line L27 (-10, -53) -> (-10, -87)
  line L28 (-10, -87) -> (-4, -87)
  line L29 (-10, -50) -> (0, -50)
  line L30 (-10, -90) -> (-10, -50)
  line L31 (0, -90) -> (-10, -90)
  line L32 (-10, -53) -> (-10, -87)
  line L33 (0, -50) -> (0, -90)
  line L34 (-4, -53) -> (-10, -53)
  line L35 (-4, -87) -> (-4, -53)
  line L36 (-108, -90) -> (-118, -90)
  line L37 (-118, -90) -> (-118, -50)
  line L38 (-118, -50) -> (-108, -50)
  line L39 (-108, -50) -> (-108, -90)
  line L40 (-108, -87) -> (-114, -87)
  line L41 (-114, -87) -> (-114, -53)
  line L42 (-114, -53) -> (-108, -53)
  line L43 (-108, -53) -> (-108, -87)
  line L44 (-10, -90) -> (-108, -90)
  line L45 (-108, -90) -> (-108, -50)
  line L46 (-108, -50) -> (-10, -50)
  line L47 (-10, -50) -> (-10, -90)
  dimension "d31" = 10
  dimension "d32" = 40
  dimension "d33" = 3
  dimension "d34" = 4
  dimension "d35" = 3
  dimension "d36" = 10
  dimension "d37" = 40
  dimension "d38" = 3
  dimension "d39" = 4
  dimension "d40" = 3
  dimension "d41" = 10
  dimension "d42" = 40
  dimension "d43" = 98
  dimension "d44" = 3
  dimension "d45" = 3
  dimension "d46" = 4
  constraint horizontal L9
  constraint vertical L15
  constraint horizontal L14
  constraint vertical L8
  constraint coincident L14.start L15.end
  constraint coincident L8.end L9.start
  constraint horizontal L11
  constraint vertical L10
  constraint horizontal L7
  constraint vertical L12
  constraint coincident L7.start L10.end
  constraint coincident L4.end L5.start
  constraint horizontal L20
  constraint vertical L21
  constraint horizontal L22
  constraint vertical L23
  constraint horizontal L24
  constraint vertical L25
  constraint horizontal L26
  constraint vertical L27
  constraint coincident L21 L24.start
  constraint horizontal L31
  constraint vertical L30
  constraint horizontal L29
  constraint vertical L33
  constraint horizontal L28
  constraint vertical L35
  constraint horizontal L34
  constraint vertical L32
  constraint coincident L24.start L30
  constraint horizontal L36
  constraint vertical L37
  constraint horizontal L38
  constraint vertical L39
  constraint horizontal L40
  constraint vertical L41
  constraint horizontal L42
  constraint vertical L43
  constraint coincident L39 L40.start
  constraint horizontal L44
  constraint vertical L45
  constraint horizontal L46
  constraint vertical L47
  measures "d31" distance of L20.start L20.end
  measures "d32" distance of L20.start L22.end
  measures "d33" distance of L20 L24
  measures "d34" distance of L23 L25
  measures "d35" distance of L22 L26
  measures "d36" distance of L20.start L20.end
  measures "d37" distance of L22.end L20.start
  measures "d38" distance of L28 L31
  measures "d39" distance of L33 L35
  measures "d40" distance of L29 L34
  measures "d41" distance of L36.start L36.end
  measures "d42" distance of L36.start L38.end
  measures "d43" distance of L30 L39
  measures "d44" distance of L36 L40
  measures "d45" distance of L38 L42
  measures "d46" distance of L37 L41